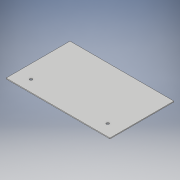
# Autodesk Inventor part: Plexiglass number plate
Saved by Autodesk Inventor 2019 (Build 230136000, 136)
## iProperties
Created: 2019-02-04
Part Number: Plexiglass number plate
Material: Generic
Document SubType Name: Modeling
Designer: mrhftc
Density: 1 g/cm^3
Appearance: Default
Author: mrhftc
Autodesk Inventor part; units mm, degrees
ref_plane "YZ Plane" through (0, 0, 0) normal (1, 0, 0) x (0, 1, 0)
ref_plane "XZ Plane" through (0, 0, 0) normal (0, 1, 0) x (-1, 0, 0)
ref_plane "XY Plane" through (0, 0, 0) normal (0, 0, 1) x (1, 0, 0)
sketch "Sketch1" plane through (0, 0, 0) normal (0, 1, 0) x (-1, 0, 0)
  line L0 (109.1682, 271.2376) -> (-55.9318, 271.2376)
  line L1 (-55.9318, 271.2376) -> (-55.9318, 169.6376)
  line L2 (-55.9318, 169.6376) -> (109.1682, 169.6376)
  line L3 (109.1682, 169.6376) -> (109.1682, 271.2376)
  circle A0 centre (87.5782, 253.2376) radius 2.1
  circle A1 centre (-34.3418, 253.2376) radius 2.1
  point P0 (0, 0)
  dimension "d4" = 4.2
  dimension "d6" = 18
  dimension "d10" = 101.6
  dimension "d13" = 165.1
  constraints: 8 end point, 2 centre point, 2 parallel, 1 horizontal, 1 perpendicular
  measures "d4" diameter of A0
  measures "d6" distance from line of L0 A0.centre
  measures "d10" distance between parallel lines of L0 L2
  measures "d13" distance between parallel lines of L1 L3
extrude "Extrusion3" add sketch "Sketch1" along normal blind 1.27
body "Solid3"
